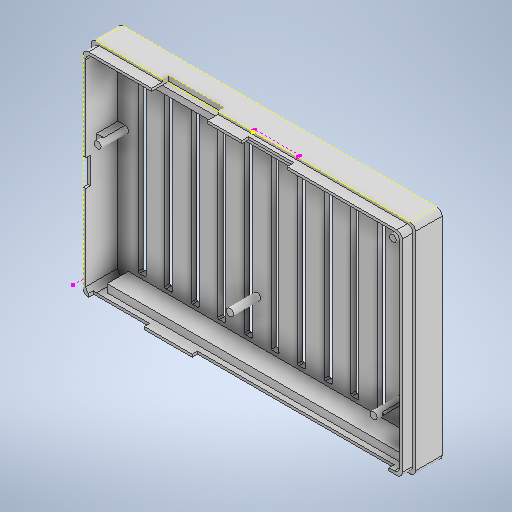
# Autodesk Inventor part: caixa_KiiRA
Saved by Autodesk Inventor 2026.3 (Build 303398000, 398)
## iProperties
Created: 2026-05-20
Part Number: caixa_KiiRA
Material: Genérico
Document SubType Name: Modeling
Designer: franciscowilke
Density: 1 g/cm^3
Appearance: Padrão
Author: franciscowilke
Autodesk Inventor part; units mm, degrees
ref_plane "YZ Plane" through (0, 0, 0) normal (1, 0, 0) x (0, 1, 0)
ref_plane "XZ Plane" through (0, 0, 0) normal (0, 1, 0) x (-1, 0, 0)
ref_plane "XY Plane" through (0, 0, 0) normal (0, 0, 1) x (1, 0, 0)
sketch "Esboço1" plane through (0, 0, 0) normal (0, 0, 1) x (1, 0, 0)
  line L0 (-59, 39) -> (59, 39)
  line L1 (59, 39) -> (59, -39)
  line L2 (59, -39) -> (-59, -39)
  line L3 (-59, -39) -> (-59, 39)
  line L4 (-59, 39) -> (59, -39) construction
  line L5 (59, 39) -> (-59, -39) construction
  line L6 (60, 40) -> (-60, 40)
  line L7 (-60, 40) -> (-60, -40)
  line L8 (-60, -40) -> (60, -40)
  line L9 (60, -40) -> (60, 40)
  line L10 (-61, 41) -> (61, 41)
  line L11 (61, 41) -> (61, -41)
  line L12 (61, -41) -> (-61, -41)
  line L13 (-61, -41) -> (-61, 41)
  point P0 (0, 0)
  dimension "d14" = 118
  dimension "d15" = 78
  dimension "d16" = 1
  dimension "d17" = 1
  constraints: 28 end point, 6 parallel, 3 perpendicular, 2 midpoint, 1 horizontal, 6 other
  measures "d14" distance of L0.start L0.end
  measures "d15" distance of L0.end L1.end
  measures "d16" distance between parallel lines of L8 L2
  measures "d17" distance between parallel lines of L12 L8
extrude "Extrusão8" add sketch "Esboço1" against normal blind 10 contours L0 L1 L2 L3 | L9 L8 L7 L6 | L10 L11 L12 L13
extrude "Extrusão9" cut sketch "Esboço1" against normal blind 8 contours L0 L1 L2 L3
extrude "Extrusão10" add sketch "Esboço1" along normal blind 4 contours L9 L8 L7 L6
fillet "Arredondamento4" radius 2 12 edges at (61, 41, -5) (60, 40, 2) (61, -41, -5) (60, -40, 2) (-61, 41, -5) (-60, 40, 2) (-60, -40, 2) (-61, -41, -5) (59, 39, -2) (-59, 39, -2) (59, -39, -2) (-59, -39, -2)
sketch "Esboço4" plane through (-59, 41, 0) normal (0, 1, 0) x (1, 0, 0)
  line L0 (120, 0) -> (120, 10) construction
  line L1 (2, -4) -> (116, -4) construction
  line L2 (75.727, -8.0038) -> (58.727, -8.0038)
  line L3 (58.727, -8.0038) -> (58.727, -1.5038)
  line L4 (58.727, -1.5038) -> (75.727, -1.5038)
  line L5 (75.727, -1.5038) -> (75.727, -8.0038)
  line L6 (45.727, -4) -> (24.727, -4)
  line L7 (24.727, -4) -> (24.727, 2.5)
  line L8 (24.727, 2.5) -> (45.727, 2.5)
  line L9 (45.727, 2.5) -> (45.727, -4)
  point P0 (59, 0)
  dimension "d46" = 6.5
  dimension "d104" = 6.5
  dimension "d105" = 17
  dimension "d107" = 21
  constraints: 16 end point, 4 parallel, 2 horizontal, 2 perpendicular, 1 point on line
  measures "d46" distance of L8.end L6.start
  measures "d104" distance of L2.end L3.end
  measures "d105" distance of L2.start L2.end
  measures "d107" distance between parallel lines of L9 L7
extrude "Extrusão11" cut sketch "Esboço4" against normal blind 4
sketch "Esboço9" plane through (-59, -41, 0) normal (0, -1, 0) x (1, 0, 0)
  line L0 (-2, 0) -> (-2, -10) construction
  line L1 (22, 2) -> (22, 4)
  line L2 (22, 4) -> (1, 4)
  line L3 (0, -10) -> (0, 0) construction
  line L4 (0, 0) -> (118, 0) construction
  line L5 (1, 0) -> (1, 4) construction
  line L6 (1, 4) -> (1, 2)
  line L7 (2, 4) -> (2, -8) construction
  line L8 (-2, 0) -> (0, 0)
  line L9 (1, 2) -> (22, 2)
  point P0 (59, 0)
  dimension "d62" = 21
  dimension "d123" = 2
  constraints: 12 end point, 3 perpendicular, 3 point on line, 1 horizontal, 1 parallel
  measures "d62" distance of L2.end L1.end
  measures "d123" distance between parallel lines of L4 L9
extrude "Extrusão14" cut sketch "Esboço9" against normal blind 6
sketch "Esboço11" plane through (-60, 38, 0) normal (-1, 0, 0) x (0, 0, 1)
  line L0 (0, -73) -> (8, -73) construction
  line L1 (4, 0) -> (4, -76) construction
  line L2 (0, 0) -> (4, 0) construction
  line L3 (0, -76) -> (0, 0) construction
  line L4 (4, -76) -> (0, -76) construction
  point P0 (0, -38)
  constraints: 1 other
sketch "Esboço12" plane through (-59, 41, -10) normal (0, 1, 0) x (1, 0, 0)
  line L0 (58.727, -10) -> (58.727, -9.0038) construction
  line L1 (58.727, -9.0038) -> (75.727, -9.0038) construction
  line L2 (75.727, -9.0038) -> (75.727, -10) construction
  line L3 (118, -10) -> (0, -10) construction
  line L4 (118, 0) -> (118, -10) construction
  line L5 (0, 0) -> (118, 0) construction
  line L6 (0, -10) -> (0, 0) construction
  line L7 (118, -10) -> (0, -10) construction
  line L8 (24.727, -10) -> (24.727, -7.5) construction
  line L9 (24.727, -7.5) -> (45.727, -7.5) construction
  line L10 (45.727, -7.5) -> (45.727, -10) construction
  line L11 (118, -10) -> (0, -10) construction
  point P0 (59, -10)
sketch "Esboço14" plane through (-61, -39, 0) normal (-1, 0, 0) x (0, 0, 1)
  line L0 (0, 78) -> (0, 0) construction
  line L1 (0, 80) -> (-10, 80) construction
  line L2 (2.326, 80) -> (2.326, 34)
  line L3 (2.326, 34) -> (6.326, 34)
  line L4 (6.326, 34) -> (6.326, 44)
  line L5 (6.326, 44) -> (2.326, 44)
  line L6 (2.326, 44) -> (2.326, 34)
  line L7 (0, 80) -> (0, 78) construction
  point P0 (0, 39)
  point P1 (2.326, 44)
  dimension "d77" = 4
  dimension "d81" = 46
  dimension "d82" = -2.326
  dimension "d108" = 10
  constraints: 10 end point, 2 parallel, 2 perpendicular, 1 point on line, 1 vertical
  measures "d77" distance of L2.end L3.end
  measures "d81" distance of L2.start L2.end
  measures "d82" distance between parallel lines of L2 L7
  measures "d108" distance between parallel lines of L3 L5
extrude "Extrusão17" cut sketch "Esboço14" against normal blind 10
sketch "Esboço16" plane through (-59, -41, 0) normal (0, -1, 0) x (1, 0, 0)
  line L0 (120, 0) -> (120, -10) construction
  line L1 (116, 4) -> (116, -8) construction
  line L2 (120, -4.0532) -> (114, -4.0532)
  line L3 (45.727, 4) -> (116, 4) construction
  line L4 (114, 2.0002) -> (40, 2.0002)
  line L5 (40, 2.0002) -> (40, 8.3282)
  line L6 (40, 8.3282) -> (114, 8.3282)
  line L7 (114, 8.3282) -> (114, 2.0002)
  line L8 (114, -4.0532) -> (114, 13.3255)
  point P0 (59, 0)
  point P1 (75.727, 4)
  dimension "d84" = 6
  dimension "d90" = 6.328
  dimension "d122" = 74
  constraints: 12 end point, 1 horizontal, 1 parallel, 1 perpendicular, 1 point on line, 1 vertical
  measures "d84" distance of L2.start L2.end
  measures "d90" distance of L6.end L4.start
  measures "d122" distance of L5.end L6.end
extrude "Extrusão18" cut sketch "Esboço16" against normal blind 10
sketch "Esboço17" plane through (0, 0, -8) normal (0, 0, 1) x (1, 0, 0)
  line L0 (59, 37) -> (59, -37) construction
  circle A0 centre (54.75, 34.75) radius 1.25
  line L1 (-59, -37) -> (-59, 37) construction
  circle A1 centre (-56.3, 9.65) radius 1.25
  line L2 (-59, 10.9) -> (-56.3, 10.9)
  line L3 (-56.3, 10.9) -> (-56.3, 8.4)
  line L4 (-56.3, 8.4) -> (-59, 8.4)
  line L5 (-59, 8.4) -> (-59, 10.9)
  line L6 (54.75, 33.5) -> (59, 33.5)
  line L7 (59, 33.5) -> (54.75, 33.5)
  line L8 (54.75, 33.5) -> (54.75, 36)
  line L9 (54.75, 36) -> (59, 36)
  line L10 (59, 36) -> (59, 33.5)
  line L11 (57, -39) -> (55, -39) construction
  line L12 (55, -39) -> (-55, -39)
  line L13 (-55, -39) -> (-55, -36)
  line L14 (-55, -36) -> (55, -36)
  line L15 (55, -36) -> (55, -39)
  line L16 (55, 36.5) -> (-55, 36.5)
  line L17 (-55, 36.5) -> (-55, 39)
  line L18 (-55, 39) -> (55, 39)
  line L19 (55, 39) -> (55, 36.5)
  line L20 (57, -39) -> (-57, -39) construction
  line L21 (-6.57, -39) -> (-6.57, -20)
  line L22 (-6.57, -20) -> (-59, -20)
  circle A2 centre (-6.57, -20) radius 1.3
  line L23 (59, -26.58) -> (47.5, -26.58)
  line L24 (47.5, -26.58) -> (47.5, -39)
  circle A3 centre (47.5, -26.58) radius 1.3
  point P0 (0, 0)
  point P1 (-56.3, 10.9)
  dimension "d99" = 2.5
  dimension "d94" = 2.5
  dimension "d102" = 2.7
  dimension "d103" = 2.5
  dimension "d124" = 110
  dimension "d126" = 3
  dimension "d127" = 110
  dimension "d128" = 2.5
  dimension "d129" = 52.43
  dimension "d131" = 2.6
  dimension "d133" = 19
  dimension "d134" = 11.5
  dimension "d135" = 12.42
  dimension "d136" = 2.6
  constraints: 42 end point, 7 perpendicular, 7 point on line, 6 parallel, 3 centre point, 3 horizontal, 2 coincident, 2 point on circle, 1 tangent, 3 other
  measures "d94" diameter of A0
  measures "d102" distance of L2.start L2.end
  measures "d103" distance of L4.end L2.start
  measures "d124" distance of L13.end L14.end
  measures "d126" distance of L14.end L12.start
  measures "d127" distance of L17.end L19.start
  measures "d128" distance of L19.start L19.end
  measures "d129" distance of L21.end L22.end
  measures "d131" diameter of A2
  measures "d133" distance of L21.start L21.end
  measures "d134" distance of L23.start L23.end
  measures "d135" distance of L23.end L24.end
  measures "d136" diameter of A3
extrude "Extrusão19" add sketch "Esboço17" along normal blind 10.25 contours A0 L8 | L8 A0 | A1 L3 | L3 A1 | A2 L22 L21 | L21 L22 A2 | A3 L23 L24 | L24 L23 A3
extrude "Extrusão20" add sketch "Esboço17" along normal blind 8 contours A0 L9 L10 L6 | A1 L4 L5 L2 | L12 L24 L14 L15 | L12 L21 L14 L24 | L12 L13 L14 L21 | L16 L17 L18 L19
sketch "Esboço18" plane through (0, 0, -10) normal (0, 0, -1) x (-1, 0, 0)
  line L0 (-51.6443, 35.3553) -> (-48.6443, 35.3553)
  line L1 (-48.6443, 35.3553) -> (-48.6443, -34.6447)
  line L2 (-48.6443, -34.6447) -> (-51.6443, -34.6447)
  line L3 (-51.6443, -34.6447) -> (-51.6443, 35.3553)
  line L4 (-41.6443, 35.3553) -> (-38.6443, 35.3553)
  line L5 (-38.6443, 35.3553) -> (-38.6443, -34.6447)
  line L6 (-38.6443, -34.6447) -> (-41.6443, -34.6447)
  line L7 (-41.6443, -34.6447) -> (-41.6443, 35.3553)
  line L8 (-31.6443, 35.3553) -> (-28.6443, 35.3553)
  line L9 (-28.6443, 35.3553) -> (-28.6443, -34.6447)
  line L10 (-28.6443, -34.6447) -> (-31.6443, -34.6447)
  line L11 (-31.6443, -34.6447) -> (-31.6443, 35.3553)
  line L12 (-21.6443, 35.3553) -> (-18.6443, 35.3553)
  line L13 (-18.6443, 35.3553) -> (-18.6443, -34.6447)
  line L14 (-18.6443, -34.6447) -> (-21.6443, -34.6447)
  line L15 (-21.6443, -34.6447) -> (-21.6443, 35.3553)
  line L16 (-11.6443, 35.3553) -> (-8.6443, 35.3553)
  line L17 (-8.6443, 35.3553) -> (-8.6443, -34.6447)
  line L18 (-8.6443, -34.6447) -> (-11.6443, -34.6447)
  line L19 (-11.6443, -34.6447) -> (-11.6443, 35.3553)
  line L20 (-1.6443, 35.3553) -> (1.3557, 35.3553)
  line L21 (1.3557, 35.3553) -> (1.3557, -34.6447)
  line L22 (1.3557, -34.6447) -> (-1.6443, -34.6447)
  line L23 (-1.6443, -34.6447) -> (-1.6443, 35.3553)
  line L24 (8.3557, 35.3553) -> (11.3557, 35.3553)
  line L25 (11.3557, 35.3553) -> (11.3557, -34.6447)
  line L26 (11.3557, -34.6447) -> (8.3557, -34.6447)
  line L27 (8.3557, -34.6447) -> (8.3557, 35.3553)
  line L28 (18.3557, 35.3553) -> (21.3557, 35.3553)
  line L29 (21.3557, 35.3553) -> (21.3557, -34.6447)
  line L30 (21.3557, -34.6447) -> (18.3557, -34.6447)
  line L31 (18.3557, -34.6447) -> (18.3557, 35.3553)
  line L32 (28.3557, 35.3553) -> (31.3557, 35.3553)
  line L33 (31.3557, 35.3553) -> (31.3557, -34.6447)
  line L34 (31.3557, -34.6447) -> (28.3557, -34.6447)
  line L35 (28.3557, -34.6447) -> (28.3557, 35.3553)
  line L36 (38.3557, 35.3553) -> (41.3557, 35.3553)
  line L37 (41.3557, 35.3553) -> (41.3557, -34.6447)
  line L38 (41.3557, -34.6447) -> (38.3557, -34.6447)
  line L39 (38.3557, -34.6447) -> (38.3557, 35.3553)
  line L40 (48.3557, 35.3553) -> (51.3557, 35.3553)
  line L41 (51.3557, 35.3553) -> (51.3557, -34.6447)
  line L42 (51.3557, -34.6447) -> (48.3557, -34.6447)
  line L43 (48.3557, -34.6447) -> (48.3557, 35.3553)
  point P0 (0, 0)
  dimension "d109" = 70
  dimension "d110" = 3
  dimension "d113" = 10
  constraints: 88 end point, 2 horizontal, 2 parallel, 1 collinear, 1 perpendicular, 79 other
  measures "d109" distance of L0.end L1.end
  measures "d110" distance of L0.start L0.end
  measures "d113" distance of L0.start L4.start
extrude "Extrusão21" cut sketch "Esboço18" against normal blind 10
fillet "Arredondamento5" radius 0.5 43 edges at (48.6443, 35.3553, -9) (38.6443, 35.3553, -9) (28.6443, 35.3553, -9) (18.6443, 35.3553, -9) (8.6443, 35.3553, -9) (-1.3557, 35.3553, -9) (-11.3557, 35.3553, -9) (-21.3557, 35.3553, -9) (-31.3557, 35.3553, -9) (-41.3557, 35.3553, -9) (-51.3557, 35.3553, -9) (51.6443, 35.3553, -9) (41.6443, 35.3553, -9) (31.6443, 35.3553, -9) (21.6443, 35.3553, -9) (11.6443, 35.3553, -9) (1.6443, 35.3553, -9) (-8.3557, 35.3553, -9) (-18.3557, 35.3553, -9) (-28.3557, 35.3553, -9) (-38.3557, 35.3553, -9) (-48.3557, 35.3553, -9) (51.6443, -34.6447, -9) (41.6443, -34.6447, -9) (31.6443, -34.6447, -9) (21.6443, -34.6447, -9) (11.6443, -34.6447, -9) (1.6443, -34.6447, -9) (-8.3557, -34.6447, -9) (-18.3557, -34.6447, -9) (-48.3557, -34.6447, -9) (-38.3557, -34.6447, -9) (-28.3557, -34.6447, -9) (-51.3557, -34.6447, -9) (-41.3557, -34.6447, -9) (-31.3557, -34.6447, -9) (-21.3557, -34.6447, -9) (-11.3557, -34.6447, -9) (8.6443, -34.6447, -9) (18.6443, -34.6447, -9) (28.6443, -34.6447, -9) (38.6443, -34.6447, -9) (48.6443, -34.6447, -9)
